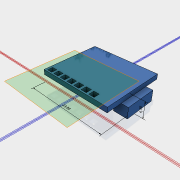
# Autodesk Inventor part: ЛЦМК0000002.00.00.00.00.03
Saved by Autodesk Inventor 2021.2 (Build 252289000, 289)
## iProperties
Created: 2025-10-23
Part Number: ЛЦМК0000002.00.00.00.00.03
Material: Типовые
Document SubType Name: Modeling
Designer: Захаров
Density: 1 g/cm^3
Appearance: С вкраплениями — сатинированная — синяя
Author: Захаров
Autodesk Inventor part; units mm, degrees
ref_plane "YZ Plane" through (0, 0, 0) normal (1, 0, 0) x (0, 1, 0)
ref_plane "XZ Plane" through (0, 0, 0) normal (0, 1, 0) x (-1, 0, 0)
ref_plane "XY Plane" through (0, 0, 0) normal (0, 0, 1) x (1, 0, 0)
ref_plane "РабПлоскость1" through (-8.75, -1.3, -1.3) normal (0, -1, 0) x (1, 0, 0)
sketch "Эскиз1" plane through (-8.75, -1.3, -1.3) normal (0, -1, 0) x (1, 0, 0)
  line L0 (21, -15.4) -> (0, -15.4)
  line L1 (0, -15.4) -> (0, 2.6)
  line L2 (0, 2.6) -> (21, 2.6)
  line L3 (21, 2.6) -> (21, -15.4)
  point P0 (8.75, 1.3)
  point P1 (0, 2.6)
  dimension "d0" = 21
  dimension "d1" = 18
  constraints: 8 end point, 2 parallel, 1 coincident, 1 horizontal, 1 perpendicular, 1 other
  measures "d0" distance of L1.end L2.end
  measures "d1" distance of L0.end L1.end
extrude "Выдавливание1" add sketch "Эскиз1" along normal blind 1.5
sketch "Эскиз2" plane through (-8.75, -2.8, -1.3) normal (0, -1, 0) x (1, 0, 0)
  line L0 (23, -10.9) -> (19, -10.9)
  line L1 (19, -10.9) -> (19, -1.9)
  line L2 (19, -1.9) -> (23, -1.9)
  line L3 (23, -1.9) -> (23, -10.9)
  line L4 (21, -15.4) -> (21, 2.6) projected
  line L5 (23, -10.9) -> (19, -1.9) construction
  line L6 (19, -10.9) -> (23, -1.9) construction
  point P0 (8.75, 1.3)
  point P1 (21, -6.4)
  dimension "d4" = 9
  dimension "d5" = 4
  constraints: 12 end point, 3 midpoint, 2 parallel, 1 horizontal, 1 perpendicular
  measures "d4" distance of L2.end L0.start
  measures "d5" distance of L1.end L2.end
extrude "Выдавливание2" add sketch "Эскиз2" along normal blind 3.2
sketch "Эскиз3" plane through (-8.75, -2.8, -1.3) normal (0, -1, 0) x (1, 0, 0)
  line L0 (2.35, 2.1) -> (2.35, 0.5)
  line L1 (0.75, 2.1) -> (2.35, 2.1)
  line L2 (0.75, 0.5) -> (0.75, 2.1)
  line L3 (2.35, 0.5) -> (0.75, 0.5)
  line L4 (4.75, 2.1) -> (4.75, 0.5)
  line L5 (3.15, 2.1) -> (4.75, 2.1)
  line L6 (3.15, 0.5) -> (3.15, 2.1)
  line L7 (4.75, 0.5) -> (3.15, 0.5)
  line L8 (7.15, 2.1) -> (7.15, 0.5)
  line L9 (5.55, 2.1) -> (7.15, 2.1)
  line L10 (5.55, 0.5) -> (5.55, 2.1)
  line L11 (7.15, 0.5) -> (5.55, 0.5)
  line L12 (9.55, 2.1) -> (9.55, 0.5)
  line L13 (7.95, 2.1) -> (9.55, 2.1)
  line L14 (7.95, 0.5) -> (7.95, 2.1)
  line L15 (9.55, 0.5) -> (7.95, 0.5)
  line L16 (11.95, 2.1) -> (11.95, 0.5)
  line L17 (10.35, 2.1) -> (11.95, 2.1)
  line L18 (10.35, 0.5) -> (10.35, 2.1)
  line L19 (11.95, 0.5) -> (10.35, 0.5)
  line L20 (14.35, 2.1) -> (14.35, 0.5)
  line L21 (12.75, 2.1) -> (14.35, 2.1)
  line L22 (12.75, 0.5) -> (12.75, 2.1)
  line L23 (14.35, 0.5) -> (12.75, 0.5)
  line L24 (16.75, 2.1) -> (16.75, 0.5)
  line L25 (15.15, 2.1) -> (16.75, 2.1)
  line L26 (15.15, 0.5) -> (15.15, 2.1)
  line L27 (16.75, 0.5) -> (15.15, 0.5)
  point P0 (8.75, 1.3)
extrude "Выдавливание3" cut sketch "Эскиз3" against normal blind 2.7
